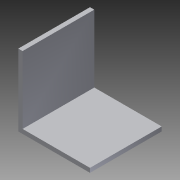
# Autodesk Inventor part: Bracket
Saved by Autodesk Inventor 2013 (Build 170138000, 138)
## iProperties
Created: 2015-07-03
Part Number: Bracket
Material: Aluminum 6061
Document SubType Name: Modeling
Designer: Kyle
Density: 2.71 g/cm^3
Mass: 0.64615 g
Surface Area: 6.82708 cm^2
Volume: 0.238432 cm^3
Author: Kyle
Autodesk Inventor part; units mm, degrees
ref_plane "YZ Plane" through (0, 0, 0) normal (1, 0, 0) x (0, 1, 0)
ref_plane "XZ Plane" through (0, 0, 0) normal (0, 1, 0) x (-1, 0, 0)
ref_plane "XY Plane" through (0, 0, 0) normal (0, 0, 1) x (1, 0, 0)
sketch "Sketch1" plane through (0, 0, 0) normal (0, 0, 1) x (1, 0, 0)
  line L0 (0, 0) -> (0, 12.7)
  line L1 (0, 0) -> (12.7, 0)
  line L2 (0.762, 12.7) -> (0.762, 0.762)
  line L3 (0.762, 0.762) -> (12.7, 0.762)
  line L4 (0.762, 12.7) -> (0, 12.7)
  line L5 (12.7, 0.762) -> (12.7, 0)
  dimension "d0" = 12.7
  dimension "d1" = 12.7
  dimension "d2" = 0.762
  constraints: 12 end point, 3 perpendicular, 1 parallel, 1 vertical, 1 other
  measures "d0" distance of L0.start L0.end
  measures "d1" distance of L0.start L1.end
  measures "d2" distance between parallel lines of L0 L2
extrude "Extrusion1" add sketch "Sketch1" along normal blind 12.7
body "Solid1"
